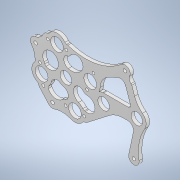
# Autodesk Inventor part: モータマウント
Saved by Autodesk Inventor 2022.2 (Build 262287030, 287C)
## iProperties
Created: 2022-03-06
Part Number: モータマウント
Material: Aluminum 2014-T6
Document SubType Name: Modeling
Designer: acps
Density: 2.78927 g/cm^3
Appearance: Satin
Author: acps
Autodesk Inventor part; units mm, degrees
ref_plane "YZ Plane" through (0, 0, 0) normal (1, 0, 0) x (0, 1, 0)
ref_plane "XZ Plane" through (0, 0, 0) normal (0, 1, 0) x (-1, 0, 0)
ref_plane "XY Plane" through (0, 0, 0) normal (0, 0, 1) x (1, 0, 0)
sketch "Sketch2" plane through (0, 0, 0) normal (0, 0, 1) x (1, 0, 0)
  circle A0 centre (57.1303, 18) radius 23.5 construction
  circle A1 centre (28.5108, 14.8066) radius 30.5 construction
  circle A2 centre (-11.7069, 38.9422) radius 15 construction
  circle A3 centre (-24.9422, 10.2931) radius 15 construction
  circle A4 centre (3.7069, -2.9422) radius 15 construction
  circle A5 centre (16.9422, 25.7069) radius 15 construction
  circle A6 centre (-19.7069, 38.9422) radius 1.25
  circle A7 centre (-3.7069, 38.9422) radius 1.25
  circle A8 centre (-23.553, 2.4146) radius 1.25
  circle A9 centre (-26.3314, 18.1716) radius 1.25
  circle A10 centre (-4.2931, -2.9422) radius 1.25
  circle A11 centre (11.7069, -2.9422) radius 1.25
  circle A12 centre (19.6783, 33.2245) radius 1.25
  circle A13 centre (14.206, 18.1894) radius 1.25
  line L0 (-19.7069, 38.9422) -> (-3.7069, 38.9422) construction
  line L1 (-23.553, 2.4146) -> (-26.3314, 18.1716) construction
  line L2 (11.7069, -2.9422) -> (-4.2931, -2.9422) construction
  line L3 (19.6783, 33.2245) -> (14.206, 18.1894) construction
  line L4 (0, 0) -> (-16.0294, 0) construction
  circle A14 centre (-11.7069, 38.9422) radius 5.5
  circle A15 centre (-24.9422, 10.2931) radius 5.5
  circle A16 centre (3.7069, -2.9422) radius 5.5
  circle A17 centre (16.9422, 25.7069) radius 5.5
  circle A18 centre (-4, 18) radius 5.005
  circle A19 centre (-15.5782, -6.2147) radius 1.5
  circle A20 centre (-30.1645, 30.8358) radius 1.5
  circle A21 centre (46.8863, 48.5466) radius 1.5
  arc A22 (-22.2098, 19.2085) -> (-30.559, 17.7363) centre (-26.3314, 18.1716) ccw
  arc A23 (-31.0997, 16.1527) -> (-28.7242, 2.6809) centre (-24.9422, 10.2931) ccw
  arc A24 (-31.0997, 16.1527) -> (-30.559, 17.7363) centre (-32.5485, 17.5315) ccw
  arc A25 (-22.2098, 19.2085) -> (-21.1601, 17.9053) centre (-20.2702, 19.6964) ccw
  arc A26 (-18.7847, 4.4335) -> (-21.1601, 17.9053) centre (-24.9422, 10.2931) ccw
  arc A27 (-27.6746, 1.3777) -> (-19.3253, 2.8499) centre (-23.553, 2.4146) ccw
  arc A28 (-27.6746, 1.3777) -> (-28.7242, 2.6809) centre (-29.6141, 0.8897) ccw
  arc A29 (-18.7847, 4.4335) -> (-19.3253, 2.8499) centre (-17.3359, 3.0547) ccw
  arc A30 (-20.0124, 43.1812) -> (-20.0124, 34.7032) centre (-19.7069, 38.9422) ccw
  arc A31 (-20.0124, 43.1812) -> (-18.5468, 43.9886) centre (-20.1561, 45.176) ccw
  arc A32 (-18.5468, 33.8957) -> (-20.0124, 34.7032) centre (-20.1561, 32.7083) ccw
  arc A33 (-4.8671, 43.9886) -> (-18.5468, 43.9886) centre (-11.7069, 38.9422) ccw
  arc A34 (-18.5468, 33.8957) -> (-4.8671, 33.8957) centre (-11.7069, 38.9422) ccw
  arc A35 (-3.4014, 34.7032) -> (-3.4014, 43.1812) centre (-3.7069, 38.9422) ccw
  arc A36 (-4.8671, 43.9886) -> (-3.4014, 43.1812) centre (-3.2577, 45.176) ccw
  arc A37 (-3.4014, 34.7032) -> (-4.8671, 33.8957) centre (-3.2577, 32.7083) ccw
  arc A38 (23.7662, 32.0617) -> (15.7995, 34.9613) centre (19.6783, 33.2245) ccw
  arc A39 (10.1182, 19.3521) -> (18.0849, 16.4525) centre (14.206, 18.1894) ccw
  arc A40 (14.5394, 33.8602) -> (9.8607, 21.0055) centre (16.9422, 25.7069) ccw
  arc A41 (19.3449, 17.5536) -> (24.0236, 30.4083) centre (16.9422, 25.7069) ccw
  arc A42 (14.5394, 33.8602) -> (15.7995, 34.9613) centre (13.9741, 35.7787) ccw
  arc A43 (23.7662, 32.0617) -> (24.0236, 30.4083) centre (25.6899, 31.5145) ccw
  arc A44 (10.1182, 19.3521) -> (9.8607, 21.0055) centre (8.1945, 19.8993) ccw
  arc A45 (19.3449, 17.5536) -> (18.0849, 16.4525) centre (19.9103, 15.6351) ccw
  arc A46 (-4.5986, 1.2968) -> (-4.5986, -7.1812) centre (-4.2931, -2.9422) ccw
  arc A47 (10.5468, 2.1043) -> (-3.1329, 2.1043) centre (3.7069, -2.9422) ccw
  arc A48 (-3.1329, -7.9886) -> (10.5468, -7.9886) centre (3.7069, -2.9422) ccw
  arc A49 (12.0124, -7.1812) -> (12.0124, 1.2968) centre (11.7069, -2.9422) ccw
  arc A50 (-4.5986, 1.2968) -> (-3.1329, 2.1043) centre (-4.7423, 3.2917) ccw
  arc A51 (-3.1329, -7.9886) -> (-4.5986, -7.1812) centre (-4.7423, -9.176) ccw
  arc A52 (10.5468, 2.1043) -> (12.0124, 1.2968) centre (12.1561, 3.2917) ccw
  arc A53 (12.0124, -7.1812) -> (10.5468, -7.9886) centre (12.1561, -9.176) ccw
  circle A54 centre (-30.1645, 30.8358) radius 4.5
  circle A55 centre (-15.5782, -6.2147) radius 4.5
  circle A56 centre (46.8863, 48.5466) radius 4.5
  arc A57 (-30.5814, 18.1832) -> (-33.8099, 28.1973) centre (-47.5813, 18.23) ccw
  arc A58 (-14.6344, 30.9622) -> (-22.8052, 20.544) centre (-17.0311, 24.4287) ccw
  arc A59 (-30.9013, 35.2751) -> (-23.5339, 40.7907) centre (-32.5384, 45.1401) ccw
  line L5 (-19.7069, 38.9422) -> (-26.3314, 18.1716) construction
  line L6 (-37.3099, 33.1147) -> (-23.0191, 28.5569) construction
  line L7 (-26.7349, -0.4028) -> (-18.9473, -9.1979)
  line L8 (-23.553, 2.4146) -> (-4.2931, -2.9422) construction
  arc A60 (-19.1717, 2.2612) -> (-7.3197, 0.0415) centre (-12.4976, 5.146) ccw
  line L9 (-17.2333, -12.1656) -> (-13.923, -0.2638) construction
  arc A61 (0.4406, -10.7895) -> (-14.0476, -10.4464) centre (-7.2449, -29.2539) ccw
  circle A62 centre (-4, 18) radius 8.005
  arc A63 (-11.1987, 21.5012) -> (-14.8803, 31.0568) centre (-17.4936, 24.5629) ccw
  arc A64 (-4.8671, 33.8957) -> (-1.9826, 25.7466) centre (-0.6674, 30.7972) ccw
  arc A65 (-21.1601, 17.9053) -> (-11.2582, 21.3762) centre (-17.9005, 24.466) ccw
  arc A66 (-8.7557, 11.5608) -> (-16.621, 8.5589) centre (-11.7261, 7.5388) ccw
  arc A67 (-3.0076, 2.2698) -> (-5.8203, 10.2047) centre (-6.9573, 5.3357) ccw
  arc A68 (3.1987, 14.4988) -> (6.8803, 4.9432) centre (9.4936, 11.4371) ccw
  arc A69 (-1.9826, 25.7466) -> (9.8082, 30.3282) centre (0.7402, 36.2022) ccw
  arc A70 (10.9513, 15.4564) -> (3.1987, 14.4988) centre (7.3857, 12.4623) ccw
  arc A71 (9.8082, 30.3282) -> (-0.1132, 36.6733) centre (4.866, 33.5296) ccw
  line L10 (33.4093, 8.4753) -> (14.3076, -6.3036)
  arc A72 (9.8484, 2.9342) -> (14.3427, 13.9416) centre (14.5521, 7.4349) ccw
  circle A73 centre (28.5108, 14.8066) radius 5.005
  circle A74 centre (28.5108, 14.8066) radius 8.005
  circle A75 centre (57.1303, 18) radius 5.005
  circle A76 centre (57.1303, 18) radius 8.005
  line L11 (46.8863, 39.1497) -> (46.8863, 57.9435) construction
  line L12 (40.1087, 44.2659) -> (46.8863, 39.1497) construction
  line L13 (46.8863, 39.1497) -> (58.2251, 44.6417) construction
  line L14 (43.5516, 45.4257) -> (47.0027, 42.8206) construction
  line L15 (48.1829, 44.1746) -> (52.7703, 46.3965) construction
  line L16 (-24.9279, 32.4454) -> (-26.8947, 26.2784) construction
  arc A77 (-2.3827, 42.9806) -> (43.9855, 51.9869) centre (12.7261, 89.0588) ccw
  line L17 (32.7639, 36.7063) -> (48.8479, 44.4967)
  arc A78 (32.7639, 36.7063) -> (25.4377, 25.43) centre (38.4308, 25.0064) ccw
  circle A79 centre (54.5656, -13.2323) radius 1.5
  circle A80 centre (54.5656, -13.2323) radius 4.5
  line L18 (51.8001, -4.8875) -> (54.5656, -13.2323) construction
  line L19 (60.7867, -6.9804) -> (51.8001, -4.8875) construction
  line L20 (51.8001, -4.8875) -> (45.9798, -11.7703) construction
  line L21 (48.6212, -13.2927) -> (52.198, -9.063) construction
  line L22 (54.5144, -8.5999) -> (62.1587, -10.3802) construction
  arc A81 (47.4922, 37.6274) -> (40.5866, 40.4952) centre (42.7661, 35.9953) ccw
  line L23 (47.4922, 37.6274) -> (51.6926, 25.4644)
  arc A82 (49.8021, 22.8116) -> (51.6926, 25.4644) centre (49.8021, 24.8116) ccw
  line L24 (49.8021, 22.8116) -> (28.5108, 22.8116)
  arc A83 (45.6478, 12.657) -> (33.4093, 8.4753) centre (45.6478, -7.343) ccw
  line L25 (45.6478, 12.657) -> (49.2466, 12.657)
  arc A84 (54.1398, 6.6291) -> (49.2466, 12.657) centre (49.2466, 7.657) ccw
  line L26 (54.1398, 6.6291) -> (50.1618, -12.3071)
  arc A85 (50.932, 46.5763) -> (52.0992, 41.6469) centre (54.5282, 44.8249) ccw
  arc A86 (52.7752, 40.7107) -> (52.0992, 41.6469) centre (50.8847, 40.0578) ccw
  line L27 (52.7752, 40.7107) -> (55.1732, 33.7666)
  line L28 (51.6748, 40.8337) -> (52.8996, 37.2868) construction
  arc A87 (55.1732, 33.7666) -> (61.9746, 24.3728) centre (74.0777, 40.295) ccw
  arc A88 (25.4377, 25.43) -> (28.5108, 22.8116) centre (28.018, 25.3459) ccw
  arc A89 (63.9853, 13.8662) -> (59.0017, -12.4767) centre (96.9503, -6.013) ccw
  line L29 (60.0747, 5.696) -> (58.0202, -4.0838) construction
  arc A90 (-19.3253, 2.8499) -> (-19.1717, 2.2612) centre (-17.3359, 3.0547) ccw
  point P0 (-15.3183, -1.5555)
  point P1 (-7.7694, -5.3871)
  point P2 (-11.8974, -3.6259)
  point P3 (12.8307, 1.1565)
  point P4 (27.7639, 22.7767)
  point P5 (24.4372, 21.6976)
  point P6 (-14.7584, 31.0064)
  dimension "d87" = 2.5
  dimension "d88" = 2.5
  dimension "d89" = 2.5
  dimension "d90" = 2.5
  dimension "d91" = 2.5
  dimension "d92" = 2.5
  dimension "d93" = 2.5
  dimension "d94" = 2.5
  dimension "d95" = 16
  dimension "d96" = 16
  dimension "d97" = 16
  dimension "d98" = 16
  dimension "d99" = 100
  dimension "d100" = 11
  dimension "d101" = 11
  dimension "d102" = 11
  dimension "d103" = 11
  dimension "d104" = 3
  dimension "d105" = 3
  dimension "d106" = 3
  dimension "d107" = 2
  dimension "d108" = 2
  dimension "d109" = 3
  dimension "d110" = 3
  dimension "d111" = 3
  dimension "d112" = 2
  dimension "d113" = 2
  dimension "d114" = 3
  dimension "d115" = 3
  dimension "d116" = 2
  dimension "d117" = 2
  dimension "d118" = 3
  dimension "d119" = 3
  dimension "d120" = 2
  dimension "d121" = 2
  dimension "d122" = 3
  dimension "d123" = 2
  dimension "d124" = 2
  dimension "d125" = 3
  dimension "d126" = 3
  dimension "d127" = 3
  dimension "d128" = 3
  dimension "d129" = 2
  dimension "d130" = 2
  dimension "d131" = 3
  dimension "d132" = 3
  dimension "d133" = 3
  dimension "d134" = 3
  dimension "d135" = 2
  dimension "d136" = 2
  dimension "d137" = 2
  dimension "d138" = 2
  dimension "d139" = 3
  dimension "d140" = 3
  dimension "d141" = 3
  dimension "d142" = 20
  dimension "d143" = 17
  dimension "d144" = 10
  dimension "d145" = 5
  dimension "d146" = 5
  dimension "d147" = 7
  dimension "d148" = 7
  dimension "d149" = 10.01
  dimension "d150" = 3
  constraints: 165 point on circle, 109 tangent, 91 centre point, 58 end point, 16 concentric, 12 coincident, 10 midpoint, 8 parallel, 5 horizontal, 2 perpendicular, 2 point on line, 1 vertical, 15 other
  measures "d87" diameter of A6
  measures "d88" diameter of A7
  measures "d89" diameter of A8
  measures "d90" diameter of A9
  measures "d91" diameter of A10
  measures "d92" diameter of A11
  measures "d93" diameter of A12
  measures "d94" diameter of A13
  measures "d95" distance of L0.start L0.end
  measures "d96" distance of L1.start L1.end
  measures "d97" distance of L2.start L2.end
  measures "d98" distance of L3.start L3.end
  measures "d99" angle of L4 L1
  measures "d100" diameter of A14
  measures "d101" diameter of A15
  measures "d102" diameter of A16
  measures "d103" diameter of A17
  measures "d104" diameter of A19
  measures "d105" diameter of A20
  measures "d106" diameter of A21
  measures "d107" radius of A24
  measures "d108" radius of A25
  measures "d109" radial gap between concentric circles of A15 A23
  measures "d110" radial gap between concentric circles of A15 A26
  measures "d111" radial gap between concentric circles of A22 A9
  measures "d112" radius of A29
  measures "d113" radius of A28
  measures "d114" radial gap between concentric circles of A8 A27
  measures "d115" radial gap between concentric circles of A6 A30
  measures "d116" radius of A31
  measures "d117" radius of A32
  measures "d118" radial gap between concentric circles of A14 A33
  measures "d119" radial gap between concentric circles of A34 A14
  measures "d120" radius of A36
  measures "d121" radius of A37
  measures "d122" radial gap between concentric circles of A7 A35
  measures "d123" radius of A42
  measures "d124" radius of A43
  measures "d125" radial gap between concentric circles of A38 A12
  measures "d126" radial gap between concentric circles of A13 A39
  measures "d127" radial gap between concentric circles of A17 A40
  measures "d128" radial gap between concentric circles of A41 A17
  measures "d129" radius of A44
  measures "d130" radius of A45
  measures "d131" radial gap between concentric circles of A16 A47
  measures "d132" radial gap between concentric circles of A48 A16
  measures "d133" radial gap between concentric circles of A11 A49
  measures "d134" radial gap between concentric circles of A10 A46
  measures "d135" radius of A50
  measures "d136" radius of A51
  measures "d137" radius of A52
  measures "d138" radius of A53
  measures "d139" radial gap between concentric circles of A20 A54
  measures "d140" radial gap between concentric circles of A19 A55
  measures "d141" radial gap between concentric circles of A21 A56
  measures "d142" radius of A61
  measures "d143" radius of A57
  measures "d144" radius of A59
  measures "d145" radius of A66
  measures "d146" radius of A67
  measures "d147" radius of A68
  measures "d148" radius of A63
  measures "d149" diameter of A73
  measures "d150" radial gap between concentric circles of A73 A74
extrude "Extrusion1" add sketch "Sketch2" against normal blind 3 contours A25 A26 A29 A27 A28 A23 A24 A22 | A22 A57 A54 A59 A30 A32 A34 A63 A58 | A65 A62 A66 A26 | A58 A34 A64 A62 A63 | A62 | A54 | A34 A32 A30 A31 A33 A36 A35 A37 | A69 A40 A44 A39 A70 A62 | A90 A60 A55 L7 A27 | A62 A68 A47 A67 | A71 A35 A77 A56 L17 A78 A41 A43 A38 A42 A40 | A40 A42 A38 A43 A41 A74 A45 A39 A44 | A47 A52 A49 A53 A48 A51 A46 A50 | A55 | A60 A46 A51 A48 A61 A55 | A39 A45 A41 A74 L10 A49 A72 | A56 | A56 A85 A86 L27 A87 A76 A82 L23 A81 L17 | A74 A41 A88 | A74 L24 A82 A76 A84 L25 A83 | A74 A41 | A76 | A76 A89 A80 L26 A84 | A80 picked at (21.9184, 17.0296)
body "Solid1"
